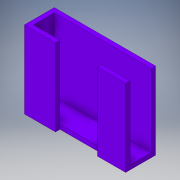
# Autodesk Inventor part: Base_Arduino
Saved by Autodesk Inventor 2019 (Build 230136000, 136)
## iProperties
Created: 2020-02-05
Part Number: Base_Arduino
Material: Generic
Document SubType Name: Modeling
Designer: Omar
Density: 1 g/cm^3
Appearance: Default
Author: Omar
Autodesk Inventor part; units mm, degrees
ref_plane "YZ Plane" through (0, 0, 0) normal (1, 0, 0) x (0, 1, 0)
ref_plane "XZ Plane" through (0, 0, 0) normal (0, 1, 0) x (-1, 0, 0)
ref_plane "XY Plane" through (0, 0, 0) normal (0, 0, 1) x (1, 0, 0)
sketch "Sketch1" plane through (0, 0, 0) normal (0, 1, 0) x (-1, 0, 0)
  line L0 (0, 0) -> (69, 0)
  line L1 (69, 0) -> (69, -15)
  line L2 (69, -15) -> (0, -15)
  line L3 (0, -15) -> (0, 0)
  dimension "d0" = 69
  dimension "d1" = 15
  constraints: 8 end point, 2 parallel, 1 horizontal, 1 perpendicular
  measures "d0" distance of L1.end L2.end
  measures "d1" distance of L0.end L1.end
extrude "Extrusion1" add sketch "Sketch1" along normal blind 3.18
sketch "Sketch2" plane through (0, 0, 0) normal (0, 1, 0) x (-1, 0, 0)
  line L0 (69, 0) -> (0, 0) projected
  line L1 (0, 0) -> (0, -15) projected
  line L2 (0, -15) -> (69, -15) projected
  line L3 (69, -15) -> (69, 0) projected
  line L4 (0, -15) -> (72.18, -15)
  line L5 (72.18, -15) -> (72.18, -18.18)
  line L6 (72.18, -18.18) -> (0, -18.18)
  line L7 (0, -18.18) -> (0, -15)
  line L8 (72.18, -15) -> (69, -15)
  line L9 (69, -15) -> (69, 0)
  line L10 (69, 0) -> (72.18, 0)
  line L11 (72.18, 0) -> (72.18, -15)
  line L12 (0, 0) -> (20, 0)
  line L13 (20, 0) -> (20, 3.18)
  line L14 (20, 3.18) -> (0, 3.18)
  line L15 (0, 3.18) -> (0, 0)
  line L16 (20, 0) -> (50, 0)
  line L17 (50, 0) -> (50, 3.18)
  line L18 (20, 3.18) -> (20, 0)
  line L19 (50, 3.18) -> (72.18, 3.18)
  line L20 (72.18, 3.18) -> (72.18, 0)
  line L21 (72.18, 0) -> (50, 0)
  line L22 (50, 0) -> (50, 3.18)
  dimension "d4" = 72.18
  dimension "d5" = 3.18
  dimension "d6" = 20
  dimension "d7" = 3.18
  dimension "d9" = 22.18
  constraints: 38 end point, 9 parallel, 5 horizontal, 5 perpendicular, 1 point on line
  measures "d4" distance of L5.end L6.end
  measures "d5" distance of L4.end L5.end
  measures "d6" distance of L14.end L13.end
  measures "d7" distance of L13.end L12.end
  measures "d9" distance of L17.end L19.end
extrude "Extrusion2" add sketch "Sketch2" along normal blind 55 contours L10 L11 L4 L3 | L0 L17 L19 L20 L10 | L4 L5 L6 L7 L2 | L0 L15 L14 L13
body "Solid1"
